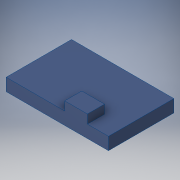
# Autodesk Inventor part: Power Booster
Saved by Autodesk Inventor 2018 (Build 220112000, 112)
## iProperties
Created: 2017-05-31
Part Number: Power Booster
Material: ABS Plastic
Document SubType Name: Modeling
Designer: Rishi
Density: 1.06 g/cm^3
Appearance: Smooth - White
Author: Rishi
Autodesk Inventor part; units mm, degrees
ref_plane "YZ Plane" through (0, 0, 0) normal (1, 0, 0) x (0, 1, 0)
ref_plane "XZ Plane" through (0, 0, 0) normal (0, 1, 0) x (-1, 0, 0)
ref_plane "XY Plane" through (0, 0, 0) normal (0, 0, 1) x (1, 0, 0)
sketch "Sketch1" plane through (0, 0, 0) normal (0, 1, 0) x (-1, 0, 0)
  line L0 (36, 23) -> (0, 23)
  line L1 (0, 23) -> (0, 0)
  line L2 (0, 0) -> (36, 0)
  line L3 (36, 0) -> (36, 23)
  dimension "d0" = 36
  dimension "d1" = 23
  constraints: 8 end point, 2 parallel, 1 horizontal, 1 perpendicular
  measures "d0" distance of L0.start L0.end
  measures "d1" distance of L2.end L0.start
extrude "Extrusion1" add sketch "Sketch1" along normal blind 4.4
sketch "Sketch2" plane through (0, 4.4, 0) normal (0, 1, 0) x (1, 0, 0)
  line L0 (-36, -23) -> (0, -23) projected
  line L1 (-15.4, -17) -> (-7.4, -17)
  line L2 (-7.4, -17) -> (-7.4, -23)
  line L3 (-7.4, -23) -> (-15.4, -23)
  line L4 (-15.4, -23) -> (-15.4, -17)
  line L5 (0, -23) -> (0, 0) projected
  dimension "d4" = 8
  dimension "d5" = 6
  dimension "d6" = 7.4
  constraints: 8 end point, 2 parallel, 1 horizontal, 1 perpendicular, 1 point on line
  measures "d4" distance of L1.start L1.end
  measures "d5" distance of L3.end L1.start
  measures "d6" distance between parallel lines of L5 L2
extrude "Extrusion2" add sketch "Sketch2" along normal blind 3.1
body "Solid1"
